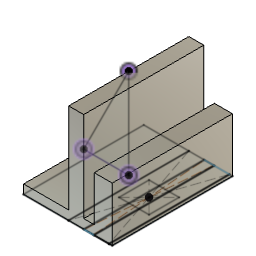
Table_Slider (Autodesk Fusion 360 design; units mm, degrees)
Autodesk Fusion 360 part; units mm, degrees
note: some values were not read from the file. Set by a fixed rule: which sketch regions a step uses.
sketch "Sketch1" plane through (0, 0, 0) normal (0, 0, 1) x (1, 0, 0)
  line L0 (6.75, 20) -> (-6.75, 20)
  line L1 (-6.75, 20) -> (-6.75, -20)
  line L2 (-6.75, -20) -> (6.75, -20)
  line L3 (6.75, -20) -> (6.75, 20)
  line L4 (6.75, 20) -> (-6.75, -20) construction
  line L5 (-6.75, 20) -> (6.75, -20) construction
  line L6 (1.5, -20) -> (-1.5, -20)
  line L7 (-1.5, -20) -> (-1.5, 20)
  line L8 (-1.5, 20) -> (1.5, 20)
  line L9 (1.5, 20) -> (1.5, -20)
  line L10 (1.5, -20) -> (-1.5, 20) construction
  line L11 (-1.5, -20) -> (1.5, 20) construction
  line L12 (1.75, -20) -> (-1.75, -20)
  line L13 (-1.75, -20) -> (-1.75, 20)
  line L14 (-1.75, 20) -> (1.75, 20)
  line L15 (1.75, 20) -> (1.75, -20)
  line L16 (1.75, -20) -> (-1.75, 20) construction
  line L17 (-1.75, -20) -> (1.75, 20) construction
  line L18 (5, -5) -> (-5, -5)
  line L19 (-5, -5) -> (-5, 5)
  line L20 (-5, 5) -> (5, 5)
  line L21 (5, 5) -> (5, -5)
  line L22 (5, -5) -> (-5, 5) construction
  line L23 (-5, -5) -> (5, 5) construction
  line L24 (1.75, -20) -> (6.75, -20)
  line L25 (6.75, -20) -> (6.75, 20)
  line L26 (6.75, 20) -> (1.75, 20)
  line L27 (1.75, 20) -> (1.75, -20)
  line L28 (-6.75, -20) -> (-21.75, -20)
  line L29 (-21.75, -20) -> (-21.75, 20)
  line L30 (-21.75, 20) -> (-6.75, 20)
  line L31 (-6.75, 20) -> (-6.75, -20)
  line L32 (6.75, 20) -> (7.75, 20)
  line L33 (7.75, 20) -> (7.75, -20)
  line L34 (7.75, -20) -> (6.75, -20)
  line L35 (6.75, -20) -> (6.75, 20)
  dimension "d1" = 13.5
  dimension "d2" = 40
  dimension "d3" = 3
  dimension "d4" = 3.5
  dimension "d5" = 40
  dimension "d6" = 10
  dimension "d7" = 10
  dimension "d18" = 5
  dimension "d19" = 15
  dimension "d20" = 40
  dimension "d29" = 1
  dimension "d30" = 40
  constraint horizontal L0
  constraint perpendicular L0 L1
  constraint parallel L0 L2
  constraint parallel L1 L3
  constraint coincident L4 origin
  constraint coincident L5 origin
  constraint horizontal L6
  constraint perpendicular L6 L7
  constraint parallel L6 L8
  constraint parallel L7 L9
  constraint coincident L10 origin
  constraint coincident L11 origin
  constraint horizontal L12
  constraint perpendicular L12 L13
  constraint parallel L12 L14
  constraint parallel L13 L15
  constraint coincident L16 origin
  constraint coincident L17 origin
  constraint horizontal L18
  constraint perpendicular L18 L19
  constraint parallel L18 L20
  constraint parallel L19 L21
  constraint coincident L22 origin
  constraint coincident L23 origin
  constraint horizontal L24
  constraint vertical L25
  constraint horizontal L26
  constraint vertical L27
  constraint horizontal L28
  constraint vertical L29
  constraint horizontal L30
  constraint vertical L31
  constraint horizontal L32
  constraint vertical L33
  constraint horizontal L34
  constraint vertical L35
  measures "d1" distance of L1.end L2.end
  measures "d2" distance of L0.end L1.end
  measures "d3" distance of L7.end L8.end
  measures "d4" distance of L13.end L14.end
  measures "d5" distance of L12.end L13.end
  measures "d6" distance of L19.end L20.end
  measures "d7" distance of L18.end L19.end
  measures "d18" distance of L12.start L2.end
  measures "d19" distance of L1.end L28.end
  measures "d20" distance of L1.end L0.end
  measures "d29" distance of L0.start L32.end
  measures "d30" distance of L0.start L2.end
extrude "Extrude1" add sketch "Sketch1" along normal blind 20 contours L0 L2 L3 L15 L18 L20 L21 L24 L25 L26 L27 L35 | L15 L18 L20 L21 L27 | L0 L1 L2 L13 L18 L19 L20 L31 | L13 L18 L19 L20 makes body 1 at (-1.75, -6.6667, 6.6667) makes body 2 at (6.75, -6.6667, 6.6667)
extrude "Extrude2" add 1 faces at (-3.4167, -6.6667, 20) along direction (0, 0, 1) blind 15 on bodies 1 bodies 1
extrude "Extrude3" add sketch "Sketch1" along normal blind 5 contours L0 L9 L14 L15 L20 L27 | L0 L7 L8 L9 L14 L20 | L9 L15 L18 L20 L27 | L2 L9 L12 L15 L18 L27 | L0 L7 L13 L14 L20 | L7 L9 L18 L20 | L2 L6 L7 L9 L12 L18 | L7 L13 L18 L20 | L2 L7 L12 L13 L18 bodies 1 2
extrude "Extrude4" add sketch "Sketch1" along normal blind 5 contours L0 L2 L3 L15 L18 L20 L21 L24 L25 L26 L27 L35 | L0 L9 L14 L15 L20 L27 | L0 L7 L8 L9 L14 L20 | L2 L9 L12 L15 L18 L27 | L0 L7 L13 L14 L20 | L2 L6 L7 L9 L12 L18 | L0 L1 L2 L13 L18 L19 L20 L31 | L2 L7 L12 L13 L18 bodies 1
extrude "Extrude5" add sketch "Sketch1" along normal blind 5 contours L15 L18 L20 L21 L27 bodies 1
extrude "Extrude6" add sketch "Sketch1" along normal blind 3 contours L1 L28 L29 L30 L31 bodies 1
extrude "Extrude7" cut 1 faces at (0.5833, -6.6667, 5) along direction (0, 0, -1) blind 2 on bodies 1 bodies 1
extrude "Extrude8" cut 1 faces at (5.0833, 6.6667, 20) along direction (0, 0, -1) blind 2 on bodies 1 bodies 1
extrude "Extrude9" cut 1 faces at (-3.4167, -6.6667, 35) along direction (0, 0, -1) blind 2 on bodies 1 bodies 1
extrude "Extrude10" add sketch "Sketch1" along normal blind 18 contours L3 L25 L32 L33 L34 L35 bodies 1
sketch "Sketch2" plane through (0, 0, 0) normal (0, 1, 0) x (1, 0, 0)
  line L0 (-21.75, -3) -> (-6.75, -33)
  line L1 (-6.75, -3) -> (-21.75, -3)
  line L2 (-6.75, -33) -> (-6.75, -3)
  line L3 (-21.75, -3) -> (-6.75, -3)
  point P0 (-21.75, -3)
  point P1 (-6.75, -33)
  point P2 (-6.75, -3)
  point P3 (-6.75, -3)
  constraint coincident P0 L0.start
  constraint coincident P1 L0.end
  constraint coincident P3 P2
extrude "Extrude11" add sketch "Sketch2" along normal blind 2.5 bodies 1
extrude "Extrude12" add sketch "Sketch2" against normal blind 2.5 bodies 1
equation "d1 = 3 mm + 0.5 mm + 5 mm + 5 mm"
equation "d8 = 5 mm + 15 mm"
equation "d31 = 3 mm + 15 mm"
